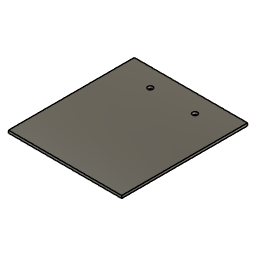
Base Plate Dimensions v2 (Autodesk Fusion 360 design; units mm, degrees)
Autodesk Fusion 360 part; units mm, degrees
sketch "Sketch1" plane through (0, 0, 0) normal (0, 0, 1) x (1, 0, 0)
  line L0 (0, 0) -> (90, 0)
  line L1 (90, 0) -> (90, 100)
  line L2 (90, 100) -> (0, 100)
  line L3 (0, 100) -> (0, 0)
  line L4 (45, 100) -> (45, 0)
  line L5 (90, 50) -> (0, 50)
  line L6 (45, 85.5) -> (49, 85.5) construction
  circle A0 centre (45, 85.5) radius 3 construction
  line L7 (45, 85.5) -> (27.25, 85.5) construction
  line L8 (45, 85.5) -> (62.75, 85.5) construction
  circle A1 centre (27.25, 85.5) radius 2
  circle A2 centre (62.75, 85.5) radius 2
  dimension "d1" = 90
  dimension "d2" = 100
  dimension "d3" = 14.5
  dimension "d4" = 6
  dimension "d5" = 17.75
  dimension "d6" = 4
  constraint horizontal L0
  constraint vertical L1
  constraint horizontal L2
  constraint vertical L3
  constraint coincident L0.start L3.end
  constraint midpoint L2 L4.start
  constraint midpoint L0 L4.end
  constraint midpoint L1 L5.start
  constraint midpoint L3 L5.end
  constraint coincident L6.start A0.centre
  constraint perpendicular L4 L7
  constraint symmetric L4 L6.start A0.centre
  constraint symmetric L4 L7.end L8.end
  constraint coincident L7.end A1.centre
  constraint symmetric L4 A1 A2
  measures "d1" distance of L0.start L0.end
  measures "d2" distance of L0.start L2.end
  measures "d3" distance of L4.start L6.start
  measures "d4" diameter of A0
  measures "d5" distance of L6.start L7.end
  measures "d6" diameter of A1
extrude "Extrude1" add sketch "Sketch1" along normal blind 2
